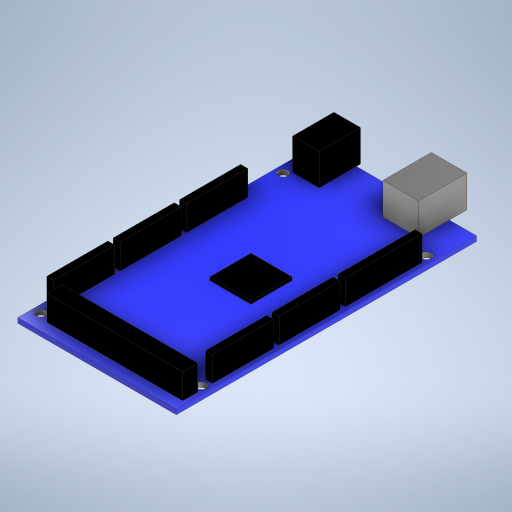
# Autodesk Inventor part: ArduinoMega
Saved by Autodesk Inventor 2024 (Build 280153000, 153)
## iProperties
Created: 2024-06-04
Part Number: ArduinoMega
Material: Genérico
Document SubType Name: Modeling
Designer: alexa
Density: 1 g/cm^3
Appearance: Valor por defecto
Author: alexa
Autodesk Inventor part; units mm, degrees
ref_plane "YZ Plane" through (0, 0, 0) normal (1, 0, 0) x (0, 1, 0)
ref_plane "XZ Plane" through (0, 0, 0) normal (0, 1, 0) x (-1, 0, 0)
ref_plane "XY Plane" through (0, 0, 0) normal (0, 0, 1) x (1, 0, 0)
sketch "Sketch1" plane through (0, 0, 0) normal (0, 1, 0) x (-1, 0, 0)
  line L0 (-26.85, 50.85) -> (26.85, 50.85)
  line L1 (26.85, 50.85) -> (26.85, -50.85)
  line L2 (26.85, -50.85) -> (-26.85, -50.85)
  line L3 (-26.85, -50.85) -> (-26.85, 50.85)
  line L4 (-26.85, 50.85) -> (26.85, -50.85) construction
  line L5 (26.85, 50.85) -> (-26.85, -50.85) construction
  point P0 (0, 0)
  dimension "d0" = 53.7
  dimension "d1" = 101.7
  constraints: 12 end point, 2 midpoint, 2 parallel, 1 horizontal, 1 perpendicular
  measures "d0" distance of L1.end L2.end
  measures "d1" distance of L0.end L1.end
extrude "Extrusion1" add sketch "Sketch1" along normal blind 1.7
sketch "Sketch2" plane through (0, 1.7, 0) normal (0, 1, 0) x (1, 0, 0)
  line L0 (26.85, 50.85) -> (-26.85, 50.85) projected
  line L1 (-26.85, 50.85) -> (-26.85, -50.85) projected
  line L2 (-22.85, 38.25) -> (-13.85, 38.25)
  line L3 (-13.85, 38.25) -> (-13.85, 52.25)
  line L4 (-13.85, 52.25) -> (-22.85, 52.25)
  line L5 (-22.85, 52.25) -> (-22.85, 38.25)
  point P0 (0, 0)
  dimension "d6" = 9
  dimension "d7" = 14
  constraints: 8 end point, 2 parallel, 1 horizontal, 1 perpendicular
  measures "d6" distance of L4.end L3.end
  measures "d7" distance of L3.end L2.end
extrude "Extrusion2" add sketch "Sketch2" along normal blind 10.7
sketch "Sketch3" plane through (0, 1.7, 0) normal (0, 1, 0) x (1, 0, 0)
  line L0 (26.85, 50.85) -> (-26.85, 50.85) projected
  line L1 (17.65, 40.45) -> (5.55, 40.45)
  line L2 (5.55, 40.45) -> (5.55, 56.85)
  line L3 (5.55, 56.85) -> (17.65, 56.85)
  line L4 (17.65, 56.85) -> (17.65, 40.45)
  point P0 (0, 0)
  dimension "d12" = 12.1
  dimension "d13" = 16.4
  constraints: 8 end point, 2 parallel, 1 horizontal, 1 perpendicular
  measures "d12" distance of L2.end L3.end
  measures "d13" distance of L1.end L2.end
extrude "Extrusion3" add sketch "Sketch3" along normal blind 10.8
sketch "Sketch4" plane through (0, 1.7, 0) normal (0, 1, 0) x (1, 0, 0)
  line L0 (-26.85, -50.85) -> (26.85, -50.85) projected
  line L1 (-26.85, 50.85) -> (-26.85, -50.85) projected
  line L2 (-20.55, -47.35) -> (25.55, -47.35)
  line L3 (25.55, -47.35) -> (25.55, -42.25)
  line L4 (25.55, -42.25) -> (-20.55, -42.25)
  line L5 (-20.55, -42.25) -> (-20.55, -47.35)
  point P0 (0, 0)
  dimension "d18" = 46.1
  dimension "d19" = 5.1
  constraints: 8 end point, 2 parallel, 1 horizontal, 1 perpendicular
  measures "d18" distance of L4.end L3.end
  measures "d19" distance of L3.end L2.end
extrude "Extrusion4" add sketch "Sketch4" along normal blind 8.5
sketch "Sketch5" plane through (0, 1.7, 0) normal (0, 1, 0) x (1, 0, 0)
  line L0 (-26.85, -50.85) -> (26.85, -50.85) projected
  line L1 (-25.55, -42.35) -> (-23.15, -42.35)
  line L2 (-23.15, -42.35) -> (-23.15, -21.65)
  line L3 (-23.15, -21.65) -> (-25.55, -21.65)
  line L4 (-25.55, -21.65) -> (-25.55, -42.35)
  line L5 (-25.55, -19.85) -> (-23.15, -19.85)
  line L6 (-23.15, -19.85) -> (-23.15, 0.85)
  line L7 (-23.15, 0.85) -> (-25.55, 0.85)
  line L8 (-25.55, 0.85) -> (-25.55, -19.85)
  line L9 (-25.55, 2.65) -> (-23.15, 2.65)
  line L10 (-23.15, 2.65) -> (-23.15, 23.35)
  line L11 (-23.15, 23.35) -> (-25.55, 23.35)
  line L12 (-25.55, 23.35) -> (-25.55, 2.65)
  line L13 (25.55, -37.25) -> (23.15, -37.25)
  line L14 (23.15, -37.25) -> (23.15, -16.55)
  line L15 (23.15, -16.55) -> (25.55, -16.55)
  line L16 (25.55, -16.55) -> (25.55, -37.25)
  line L17 (25.55, -14.75) -> (23.15, -14.75)
  line L18 (23.15, -14.75) -> (23.15, 5.95)
  line L19 (23.15, 5.95) -> (25.55, 5.95)
  line L20 (25.55, 5.95) -> (25.55, -14.75)
  line L21 (25.55, 7.75) -> (23.15, 7.75)
  line L22 (23.15, 7.75) -> (23.15, 33.75)
  line L23 (23.15, 33.75) -> (25.55, 33.75)
  line L24 (25.55, 33.75) -> (25.55, 7.75)
  point P0 (0, 0)
  dimension "d24" = 2.4
  dimension "d25" = 20.7
  dimension "d26" = 1.8
  dimension "d27" = 20.7
  dimension "d28" = 1.8
  dimension "d29" = 20.7
  dimension "d32" = 2.4
  dimension "d33" = 20.7
  dimension "d34" = 1.8
  dimension "d35" = 20.7
  dimension "d36" = 1.8
  dimension "d37" = 26
  constraints: 48 end point, 12 parallel, 6 horizontal, 6 perpendicular
  measures "d24" distance of L3.end L2.end
  measures "d25" distance of L2.end L1.end
  measures "d26" distance of L3.end L5.start
  measures "d27" distance of L6.end L5.end
  measures "d28" distance of L7.end L9.start
  measures "d29" distance of L10.end L9.end
  measures "d32" distance of L14.end L15.end
  measures "d33" distance of L13.end L14.end
  measures "d34" distance of L15.end L17.start
  measures "d35" distance of L17.end L18.end
  measures "d36" distance of L19.end L21.start
  measures "d37" distance of L21.end L22.end
extrude "Extrusion5" add sketch "Sketch5" along normal blind 8.5
sketch "Sketch6" plane through (0, 1.7, 0) normal (0, 1, 0) x (1, 0, 0)
  line L0 (-22.85, 50.85) -> (-26.85, 50.85) projected
  line L1 (-26.85, 50.85) -> (-26.85, -50.85) projected
  line L2 (-5.25, 6.55) -> (8.75, 6.55)
  line L3 (8.75, 6.55) -> (8.75, -7.45)
  line L4 (8.75, -7.45) -> (-5.25, -7.45)
  line L5 (-5.25, -7.45) -> (-5.25, 6.55)
  point P0 (0, 0)
  dimension "d42" = 14
  dimension "d43" = 14
  constraints: 8 end point, 2 parallel, 1 horizontal, 1 perpendicular
  measures "d42" distance of L3.end L4.end
  measures "d43" distance of L2.end L3.end
extrude "Extrusion6" add sketch "Sketch6" along normal blind 1
sketch "Sketch7" plane through (0, 1.7, 0) normal (0, 1, 0) x (1, 0, 0)
  circle A0 centre (-24.25, 36.5) radius 1.65
  point P0 (0, 0)
  point P1 (-26.85, 50.85)
  dimension "d48" = 3.3
  dimension "d64" = 14.35
  constraints: 1 centre point
  measures "d48" diameter of A0
  measures "d64" vertical distance of point (-26.85, 50.85) A0.centre
extrude "Extrusion7" cut sketch "Sketch7" against normal blind 2
mirror "Mirror1" about plane through (0, 0, 0) normal (1, 0, 0) of "Extrusion7"
sketch "Sketch8" plane through (0, 1.7, 0) normal (0, 1, 0) x (1, 0, 0)
  line L0 (-26.85, -50.85) -> (26.85, -50.85) projected
  line L1 (-26.85, 50.85) -> (-26.85, -50.85) projected
  circle A0 centre (-24.25, -45.65) radius 1.65
  point P0 (0, 0)
  dimension "d53" = 3.3
  dimension "d63" = 96.5
  constraints: 1 centre point
  measures "d53" diameter of A0
  measures "d63" vertical distance of L1.start A0.centre
extrude "Extrusion8" cut sketch "Sketch8" against normal blind 2
sketch "Sketch9" plane through (0, 1.7, 0) normal (0, 1, 0) x (1, 0, 0)
  line L0 (23.15, 5.95) -> (23.15, -14.75) projected
  circle A0 centre (24.25, -39.75) radius 1.65
  line L1 (23.15, -37.25) -> (25.55, -37.25) projected
  point P0 (0, 0)
  point P1 (26.85, 50.85)
  dimension "d59" = 3.3
  dimension "d60" = 2.5
  constraints: 1 centre point
  measures "d59" diameter of A0
  measures "d60" distance from line of L1 A0.centre
extrude "Extrusion9" cut sketch "Sketch9" against normal blind 2
body "Solid1"
